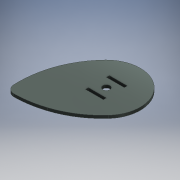
# Autodesk Inventor part: leva00
Saved by Autodesk Inventor 2016 (Build 200138000, 138)
## iProperties
Created: 2016-09-20
Part Number: leva00
Material: Madera (abedul)
Document SubType Name: Modeling
Designer: i95sa
Density: 0.55 g/cm^3
Appearance: Gris plomo - Pulido
Author: i95sa
Autodesk Inventor part; units mm, degrees
ref_plane "YZ Plane" through (0, 0, 0) normal (1, 0, 0) x (0, 1, 0)
ref_plane "XZ Plane" through (0, 0, 0) normal (0, 1, 0) x (-1, 0, 0)
ref_plane "XY Plane" through (0, 0, 0) normal (0, 0, 1) x (1, 0, 0)
sketch "Boceto1" plane through (0, 0, 0) normal (0, 0, 1) x (1, 0, 0)
  arc A0 (32.3483, 34.4474) -> (-32.3483, -34.4474) centre (0, 0) ccw
  arc A1 (-49.7814, -53.0119) -> (-64.7114, -68.9107) centre (-57.2464, -60.9613) ccw
  line L0 (-66.8727, -71.2122) -> (-74.8221, -63.7472)
  line L1 (-34.0618, 32.7541) -> (-47.3108, 45.1957)
  line L2 (-47.3108, 45.1957) -> (-74.8221, -63.7472)
  line L3 (-74.8221, -63.7472) -> (-64.1421, -21.4549)
  arc A2 (-34.0618, 32.7541) -> (-64.1421, -21.4549) centre (53.101, -51.0622) ccw
  arc A3 (-64.1421, -21.4549) -> (-68.1387, -61.4883) centre (68.2518, -54.8883) ccw
  line L4 (2.4883, 2.6498) -> (32.3483, 34.4474)
  line L5 (-2.4883, -2.6498) -> (-66.8727, -71.2122)
  arc A4 (-32.3483, -34.4474) -> (32.3483, 34.4474) centre (0, 0) ccw
  arc A5 (-64.7114, -68.9107) -> (-49.7814, -53.0119) centre (-57.2464, -60.9613) ccw
  line L6 (-66.8727, -71.2122) -> (-58.9233, -78.6772)
  line L7 (34.8282, -31.9379) -> (48.0772, -44.3796)
  line L8 (48.0772, -44.3796) -> (-58.9233, -78.6772)
  line L9 (-58.9233, -78.6772) -> (-17.3851, -65.3627)
  arc A6 (-17.3851, -65.3627) -> (34.8282, -31.9379) centre (-54.2957, 49.79) ccw
  arc A7 (-57.0885, -71.8651) -> (-17.3851, -65.3627) centre (-59.0655, 64.6707) ccw
  dimension "d0" = 94.51
  dimension "d6" = 21.81
  dimension "d7" = 10.905
  dimension "d8" = 18.175
  dimension "d9" = 43.62
  constraints: 20 end point, 20 point on circle, 8 centre point, 6 symmetric about line, 5 point on line, 4 tangent, 1 collinear, 4 other
  measures "d0" diameter of A0
  measures "d6" diameter of A1
  measures "d7" distance of L0.start L0.end
  measures "d8" distance of L1.start L1.end
  measures "d9" distance of L0.end L3.end
extrude "Extrusión2" add sketch "Boceto1" along normal blind 4 contours A4 A0 | A0 L5 A1 A3 A2 | A6 A7 A5 L5 A4 | L5 A1 | A5 L5
sketch "Boceto2" plane through (0, 0, 4) normal (0, 0, 1) x (1, 0, 0)
  line L0 (0, 0) -> (0, 12.5)
  line L1 (0, 12.5) -> (-12.5, 12.5)
  line L2 (-12.5, 12.5) -> (-12.5, 16.7)
  line L3 (-12.5, 16.7) -> (12.5, 16.7)
  line L4 (12.5, 16.7) -> (12.5, 12.5)
  line L5 (12.5, 12.5) -> (0, 12.5)
  line L6 (0, 0) -> (12.5, 0)
  line L7 (0, 0) -> (0, -12.5)
  line L8 (0, -12.5) -> (-12.5, -12.5)
  line L9 (-12.5, -12.5) -> (-12.5, -16.7)
  line L10 (-12.5, -16.7) -> (12.5, -16.7)
  line L11 (12.5, -16.7) -> (12.5, -12.5)
  line L12 (12.5, -12.5) -> (0, -12.5)
  circle A0 centre (0, 0) radius 5
  dimension "d24" = 12.5
  dimension "d25" = 12.5
  dimension "d26" = 4.2
  dimension "d27" = 25
  dimension "d28" = 10
  constraints: 26 end point, 5 perpendicular, 5 symmetric about line, 3 point on line, 1 centre point, 1 coincident, 1 parallel, 1 vertical
  measures "d24" distance of L0.start L0.end
  measures "d25" distance of L0.end L1.end
  measures "d26" distance of L1.end L2.end
  measures "d27" distance of L2.end L3.end
  measures "d28" diameter of A0
extrude "Extrusión3" cut sketch "Boceto2" against normal blind 4
